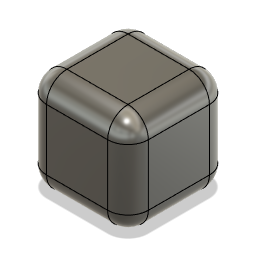
cubo v7 (Autodesk Fusion 360 design; units mm, degrees)
Autodesk Fusion 360 part; units mm, degrees
sketch "Schizzo1" plane through (0, 0, 0) normal (0, 1, 0) x (1, 0, 0)
  line L0 (0, 0) -> (-10, 0)
  line L1 (-10, 0) -> (-10, 10)
  line L2 (-10, 10) -> (0, 10)
  line L3 (0, 10) -> (0, 0)
  dimension "d1" = 10
  dimension "d2" = 10
  constraint horizontal L0
  constraint vertical L1
  constraint horizontal L2
  constraint vertical L3
  constraint coincident L0.start L3.end
  measures "d1" distance of L0.start L0.end
  measures "d2" distance of L0.start L2.end
extrude "Estrusione1" add sketch "Schizzo1" along normal blind 10
fillet "Fillet1" radius 2 12 edges at (-5, 10, 0) (-10, 10, -5) (-10, 5, 0) (-10, 5, -10) (-10, 0, -5) (-5, 0, 0) (0, 10, -5) (0, 5, 0) (-5, 0, -10) (-5, 10, -10) (0, 5, -10) (0, 0, -5)
